Autodesk Fusion 360 part; units mm, degrees
(part 2 of 2)
  constraint coincident L238 L248.end
  measures "d1" diameter of A0
  measures "d2" diameter of A1
  measures "d3" diameter of A2
  measures "d4" diameter of A3
  measures "d5" diameter of A4
  measures "d9" diameter of A111
  measures "d12" diameter of A112
extrude "Extrude1" add sketch "mriya" along normal blind 10.5 contours L201 A211 L202 A212 L203 A213 L204 A214 L205 A215 L206 A216 L207 A217 L208 A218 L209 A219 L210 A220 L211 A221 L212 A222 L213 A223 L214 A224 L215 L216 A226 L217 A227 L218 A228 L219 A229 L220 A230 L221 A231 L222 A232 L223 L224 L225 A233 L226 A234 L227 L228 L229 L230 L231 L232 L233 L234 L235 L236 L237 L238 A236 L239 L240 L241 L242 L243 L244 A237 A238 A239 A240 A241 A242 A243 A244 L245 A245 A246 A247 A248 A249 A250 A251 A252 A253 A254 L248 makes body 1
extrude "Extrude2" add sketch "mriya" along normal blind 17 contours L215 A225 L216 L237 A235 L238 L245 L248 bodies 1
extrude "Extrude3" add sketch "mriya" along normal blind 2 from surface at 1.7 contours L106 L107 L108 A113 A114 A115 L109 L110 A116 A117 L201 A211 L202 A212 L203 A213 L204 A214 L205 A215 L206 A216 L207 A217 L208 A218 L209 A219 L210 A220 L211 A221 L212 A222 L213 A223 L214 A224 L215 L216 A226 L217 A227 L218 A228 L219 A229 L220 A230 L221 A231 L222 A232 L246 L247 | L106 L107 L108 A113 A114 A115 L215 A225 L216 L246 | L109 L110 A116 A117 L215 L247 | A119 | A120 | A121 | A122 bodies 1
extrude "Extrude6" add sketch "mriya" along normal blind 1 from surface at 14.3 contours L106 L107 L108 A113 A114 A115 L215 A225 L216 L246 bodies 1
extrude "Extrude7" add sketch "mriya" along normal blind 1 from surface at 7.8 contours L109 L110 A116 A117 L215 L247 bodies 1
sketch "power-switch" plane through (-4.45, 0, 0) normal (1, 0, 0) x (0, 1, 0)
  line L0 (19.1932, 0) -> (76.4932, 0)
  line L1 (76.4932, 0) -> (76.4932, 16.8)
  line L2 (76.4932, 16.8) -> (19.1932, 16.8)
  line L3 (19.1932, 16.8) -> (19.1932, 10.5)
  line L4 (36.0932, 5.1) -> (25.6932, 5.1)
  line L5 (25.6932, 5.1) -> (25.6932, 8)
  line L6 (25.6932, 8) -> (36.0932, 8)
  line L7 (36.0932, 8) -> (36.0932, 5.1)
  line L8 (37.4932, 3.6) -> (24.2932, 3.6)
  line L9 (23.8932, 4) -> (23.8932, 9.1)
  line L10 (24.2932, 9.5) -> (37.4932, 9.5)
  line L11 (37.8932, 9.1) -> (37.8932, 4)
  line L12 (19.1932, 10.5) -> (19.1932, 0)
  line L13 (1.9932, 0) -> (76.4932, 0)
  line L14 (76.4932, 0) -> (76.4932, 17)
  line L15 (76.4932, 17) -> (19.2932, 17)
  line L16 (19.2932, 17) -> (19.2932, 10.5)
  line L17 (19.2932, 10.5) -> (1.9932, 10.5)
  line L18 (1.9932, 10.5) -> (1.9932, 0)
  arc A0 (37.8932, 9.1) -> (37.4932, 9.5) centre (37.4932, 9.1) ccw
  arc A1 (37.4932, 3.6) -> (37.8932, 4) centre (37.4932, 4) ccw
  arc A2 (23.8932, 4) -> (24.2932, 3.6) centre (24.2932, 4) ccw
  arc A3 (24.2932, 9.5) -> (23.8932, 9.1) centre (24.2932, 9.1) ccw
  constraint perpendicular L4 L5
  constraint vertical L5
  constraint perpendicular L5 L6
  constraint vertical L7
  constraint tangent L10 A0
  constraint tangent L11 A0
  constraint tangent L11 A1
  constraint tangent L8 A1
  constraint tangent L8 A2
  constraint tangent L9 A2
  constraint tangent L9 A3
  constraint tangent L10 A3
extrude "Extrude8" cut sketch "power-switch" against normal blind 2.5 contours L4 L5 L6 L7 bodies 1
extrude "Extrude9" cut sketch "power-switch" against normal blind 1 contours L8 L9 L10 L11 A0 A1 A2 A3 bodies 1
chamfer "Chamfer5" distance 0.7 angle 45 4 edges at (-6.95, 30.8932, 5.1) (-6.95, 36.0932, 6.55) (-6.95, 30.8932, 8) (-6.95, 25.6932, 6.55) on bodies 1
chamfer "Chamfer9" distance 1 angle 45 8 edges at (-4.45, 30.8932, 3.6) (-4.45, 24.0104, 3.7172) (-4.45, 23.8932, 6.55) (-4.45, 24.0104, 9.3828) (-4.45, 30.8932, 9.5) (-4.45, 37.776, 9.3828) (-4.45, 37.8932, 6.55) (-4.45, 37.776, 3.7172) on bodies 1
sketch "usb-c" plane through (0, 80.6432, 0) normal (0, 1, 0) x (-1, 0, 0)
  line L0 (3.6, 0) -> (36.1295, 0)
  line L1 (3.6, 16.7) -> (3.6, 0)
  line L2 (21.2002, 10.9) -> (21.2002, 10.1)
  arc A0 (21.2002, 10.9) -> (19.8003, 12.3) centre (19.8003, 10.9) ccw
  line L3 (11.8003, 10.1) -> (11.8003, 10.9)
  line L4 (19.8003, 8.7) -> (13.2003, 8.7)
  line L5 (21.2003, 7.3) -> (11.8002, 7.3)
  arc A1 (11.8003, 10.1) -> (13.2003, 8.7) centre (13.2003, 10.1) ccw
  line L6 (22.2003, 12.7) -> (22.2003, 8.3)
  line L7 (11.8002, 13.7) -> (21.2003, 13.7)
  arc A2 (13.2002, 12.3) -> (11.8002, 10.9) centre (13.2002, 10.9) ccw
  arc A3 (19.8003, 8.7) -> (21.2003, 10.1) centre (19.8003, 10.1) ccw
  line L8 (10.8002, 8.3) -> (10.8002, 12.7)
  line L9 (13.2002, 12.3) -> (19.8003, 12.3)
  line L10 (8.6, 0) -> (25.9, 0)
  line L11 (25.9, 10.5) -> (25.9, 16.8)
  line L12 (25.9, 16.8) -> (8.6, 16.8)
  line L13 (8.6, 16.8) -> (8.6, 0)
  line L14 (25.9, 0) -> (25.9, 10.5)
  line L15 (8.6, 0) -> (41.0881, 0)
  line L16 (41.0881, 0) -> (41.0881, 10.5)
  line L17 (41.0881, 10.5) -> (25.9, 10.5)
  line L18 (25.9, 10.5) -> (25.9, 17)
  line L19 (25.9, 17) -> (8.6, 17)
  line L20 (8.6, 17) -> (8.6, 0)
  line L21 (8.6, 0) -> (41.0881, 0)
  line L22 (41.0881, 0) -> (41.0881, 10.5)
  line L23 (41.0881, 10.5) -> (25.8, 10.5)
  line L24 (25.8, 10.5) -> (25.8, 17)
  line L25 (25.8, 17) -> (8.6, 17)
  line L26 (8.6, 17) -> (8.6, 0)
  arc A4 (11.8002, 13.7) -> (10.8002, 12.7) centre (11.8002, 12.7) ccw
  arc A5 (22.2003, 12.7) -> (21.2003, 13.7) centre (21.2003, 12.7) ccw
  arc A6 (10.8002, 8.3) -> (11.8002, 7.3) centre (11.8002, 8.3) ccw
  arc A7 (21.2003, 7.3) -> (22.2003, 8.3) centre (21.2002, 8.3) ccw
  constraint tangent L3 A2
  constraint tangent A2 L9
  constraint tangent A0 L9
  constraint tangent L2 A0
  constraint tangent L4 A3
  constraint tangent L2 A3
  constraint tangent L4 A1
  constraint tangent L3 A1
  constraint perpendicular L6 L7
  constraint perpendicular L5 L8
  constraint horizontal L5
  constraint perpendicular L5 L6
  constraint tangent L8 A4
  constraint tangent L7 A4
  constraint tangent L7 A5
  constraint tangent L6 A5
  constraint tangent L5 A6
  constraint tangent L8 A6
  constraint tangent L6 A7
  constraint tangent L5 A7
extrude "Extrude10" cut sketch "usb-c" against normal blind 2.5 contours L2 A0 L3 L4 A1 A2 A3 L9 bodies 1
extrude "Extrude11" cut sketch "usb-c" against normal blind 1 contours L5 L6 L7 L8 A4 A5 A6 A7 bodies 1
chamfer "Chamfer10" distance 1 angle 45 8 edges at (-10.8002, 80.6432, 10.5) (-11.0931, 80.6432, 13.4071) (-16.5003, 80.6432, 13.7) (-21.9074, 80.6432, 13.4071) (-22.2003, 80.6432, 10.5) (-21.9074, 80.6432, 7.5929) (-16.5002, 80.6432, 7.3) (-11.0931, 80.6432, 7.5929) on bodies 1
chamfer "Chamfer3" distance 0.9 angle 45 4 edges at (-6.95, 9.5932, 7.8) (-6.95, 53.9932, 14.3) (-7.4333, 77.6599, 14.3) (-16.1, 78.1432, 14.3) on bodies 1
chamfer "Chamfer4" distance 1 angle 45 90 edges at (-33.4441, 80.6432, 10.5) (-41.4708, 80.7193, 10.5) (-42.3594, 81.5003, 10.5) (-43.8969, 82.7148, 10.5) (-51.4665, 82.9432, 10.5) (-58.2721, 83.0196, 10.5) (-60.2606, 84.9007, 10.5) (-62.897, 87.2147, 10.5) (-73.4001, 87.4432, 10.5) (-83.9031, 87.2148, 10.5) (-86.0406, 85.4003, 10.5) (-87.5292, 84.0193, 10.5) (-94.8335, 83.9432, 10.5) (-102.9031, 83.7148, 10.5) (-107.2173, 79.7235, 10.5) (-111.045, 76.0574, 10.5) (-116.187, 75.9432, 10.5) (-121.9031, 75.7148, 10.5) (-123.4406, 74.5003, 10.5) (-124.3292, 73.7193, 10.5) (-131.4059, 73.6432, 10.5) (-141.0345, 72.4277, 10.5) (-142.25, 42.8932, 10.5) (-141.0345, 13.3587, 10.5) (-120.383, 12.1432, 10.5) (-100.9441, 12.4856, 10.5) (-96.4346, 16.5099, 10.5) (-92.7374, 19.9914, 10.5) (-84.5856, 20.1432, 10.5) (-75.6851, 19.7342, 10.5) (-70.5182, 11.4202, 10.5) (-65.1681, 2.9203, 10.5) (-56.0579, 2.4432, 10.5) (-48.3292, 2.3671, 10.5) (-47.4406, 1.5861, 10.5) (-45.9031, 0.3716, 10.5) (-37.2335, 0.1432, 10.5) (-29.3403, 0.0695, 10.5) (-28.4501, -0.712, 10.5) (-26.9041, -1.93, 10.5) (-17.1798, -2.1568, 10.5) (-5.6655, -0.9413, 10.5) (-4.45, 10.6432, 10.5) (-17.2, 80.6432, 17) (-4.45, 47.8932, 17) (-5.6655, 79.4277, 17) (-4.45, 39.2432, 0) (-5.6655, 79.4277, 0) (-24.8441, 80.6432, 0) (-41.4708, 80.7193, 0) (-42.3594, 81.5003, 0) (-43.8969, 82.7148, 0) (-51.4665, 82.9432, 0) (-58.2721, 83.0196, 0) (-60.2606, 84.9007, 0) (-62.897, 87.2147, 0) (-73.4001, 87.4432, 0) (-83.9031, 87.2148, 0) (-86.0406, 85.4003, 0) (-87.5292, 84.0193, 0) (-94.8335, 83.9432, 0) (-102.9031, 83.7148, 0) (-107.2173, 79.7235, 0) (-111.045, 76.0574, 0) (-116.187, 75.9432, 0) (-121.9031, 75.7148, 0) (-123.4406, 74.5003, 0) (-124.3292, 73.7193, 0) (-131.4059, 73.6432, 0) (-141.0345, 72.4277, 0) (-142.25, 42.8932, 0) (-141.0345, 13.3587, 0) (-120.383, 12.1432, 0) (-100.9441, 12.4856, 0) (-96.4346, 16.5099, 0) (-92.7374, 19.9914, 0) (-84.5856, 20.1432, 0) (-75.6851, 19.7342, 0) (-70.5182, 11.4202, 0) (-65.1681, 2.9203, 0) (-56.0579, 2.4432, 0) (-48.3292, 2.3671, 0) (-47.4406, 1.5861, 0) (-45.9031, 0.3716, 0) (-37.2335, 0.1432, 0) (-29.3403, 0.0695, 0) (-28.4501, -0.712, 0) (-26.9041, -1.93, 0) (-17.1798, -2.1568, 0) (-5.6655, -0.9413, 0) on bodies 1
fillet "Fillet27" radius 1.2 1 edges at (-4.45, 19.2932, 12.75) on bodies 1
chamfer "Chamfer6" distance 1 angle 45 2 edges at (-6.3, 19.2932, 17) (-5.5496, 19.2974, 17) on bodies 1
mirror "Mirror1" about plane through (0, 0, 0) normal (1, 0, 0) of bodies 1 makes body 2
named bodies: "Left", "Right"
